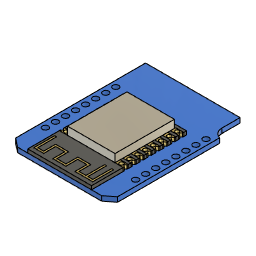
Wemos D1 Mini (Autodesk Fusion 360 design; units mm, degrees)
Autodesk Fusion 360 part; units mm, degrees
sketch "Sketch3" plane through (0, 0, 0) normal (0, 0, 1) x (1, 0, 0)
  line L0 (12.86, -17.28) -> (-12.86, -17.28)
  line L1 (-12.86, -17.28) -> (-12.86, 17.28)
  line L2 (-12.86, 17.28) -> (12.86, 17.28)
  line L3 (12.86, 17.28) -> (12.86, -17.28)
  line L4 (12.86, -17.28) -> (-12.86, 17.28) construction
  line L5 (-12.86, -17.28) -> (12.86, 17.28) construction
  line L6 (0, 55) -> (0, -53) construction
  line L7 (8.05, -17.28) -> (-8.05, -17.28)
  line L8 (-8.05, -17.28) -> (-8.05, 6.72)
  line L9 (-8.05, 6.72) -> (8.05, 6.72)
  line L10 (8.05, 6.72) -> (8.05, -17.28)
  line L11 (8.05, -17.28) -> (-8.05, 6.72) construction
  line L12 (-8.05, -17.28) -> (8.05, 6.72) construction
  line L13 (6, -9.28) -> (-6, -9.28)
  line L14 (-6, -9.28) -> (-6, 5.72)
  line L15 (6, 5.72) -> (6, -9.28)
  line L16 (6, -9.28) -> (-6, 5.72) construction
  line L17 (-6, -9.28) -> (6, 5.72) construction
  line L18 (-6, 5.72) -> (6, 5.72)
  line L19 (-9.2176, -9.28) -> (-6, -9.28) construction
  line L20 (-6, -7.98) -> (-8.05, -7.98)
  line L21 (-6, -9.28) -> (-8.05, -9.28)
  circle A0 centre (-6.9909, -8.6304) radius 0.5
  circle A1 centre (6.9909, -8.6304) radius 0.5
  line L22 (6, -9.28) -> (8.05, -9.28)
  line L23 (6, -7.98) -> (8.05, -7.98)
  arc A2 (8.05, -8.2791) -> (8.05, -8.9818) centre (8.05, -8.6304) ccw
  arc A3 (-8.05, -8.9818) -> (-8.05, -8.2791) centre (-8.05, -8.6304) ccw
  line L24 (-6, -5.98) -> (-8.05, -5.98)
  circle A4 centre (-6.9909, -6.6304) radius 0.5
  line L25 (-6, -7.28) -> (-8.05, -7.28)
  arc A5 (-8.05, -6.9818) -> (-8.05, -6.2791) centre (-8.05, -6.6304) ccw
  line L26 (6, -5.98) -> (8.05, -5.98)
  circle A6 centre (6.9909, -6.6304) radius 0.5
  arc A7 (8.05, -6.2791) -> (8.05, -6.9818) centre (8.05, -6.6304) ccw
  line L27 (6, -7.28) -> (8.05, -7.28)
  line L28 (-6, -3.98) -> (-8.05, -3.98)
  circle A8 centre (-6.9909, -4.6304) radius 0.5
  line L29 (-6, -5.28) -> (-8.05, -5.28)
  arc A9 (-8.05, -4.9818) -> (-8.05, -4.2791) centre (-8.05, -4.6304) ccw
  line L30 (6, -3.98) -> (8.05, -3.98)
  circle A10 centre (6.9909, -4.6304) radius 0.5
  arc A11 (8.05, -4.2791) -> (8.05, -4.9818) centre (8.05, -4.6304) ccw
  line L31 (6, -5.28) -> (8.05, -5.28)
  line L32 (-6, -1.98) -> (-8.05, -1.98)
  circle A12 centre (-6.9909, -2.6304) radius 0.5
  line L33 (-6, -3.28) -> (-8.05, -3.28)
  arc A13 (-8.05, -2.9818) -> (-8.05, -2.2791) centre (-8.05, -2.6304) ccw
  line L34 (6, -1.98) -> (8.05, -1.98)
  circle A14 centre (6.9909, -2.6304) radius 0.5
  arc A15 (8.05, -2.2791) -> (8.05, -2.9818) centre (8.05, -2.6304) ccw
  line L35 (6, -3.28) -> (8.05, -3.28)
  line L36 (-6, 0.02) -> (-8.05, 0.02)
  circle A16 centre (-6.9909, -0.6304) radius 0.5
  line L37 (-6, -1.28) -> (-8.05, -1.28)
  arc A17 (-8.05, -0.9818) -> (-8.05, -0.2791) centre (-8.05, -0.6304) ccw
  line L38 (6, 0.02) -> (8.05, 0.02)
  circle A18 centre (6.9909, -0.6304) radius 0.5
  arc A19 (8.05, -0.2791) -> (8.05, -0.9818) centre (8.05, -0.6304) ccw
  line L39 (6, -1.28) -> (8.05, -1.28)
  line L40 (-6, 2.02) -> (-8.05, 2.02)
  circle A20 centre (-6.9909, 1.3696) radius 0.5
  line L41 (-6, 0.72) -> (-8.05, 0.72)
  arc A21 (-8.05, 1.0182) -> (-8.05, 1.7209) centre (-8.05, 1.3696) ccw
  line L42 (6, 2.02) -> (8.05, 2.02)
  circle A22 centre (6.9909, 1.3696) radius 0.5
  arc A23 (8.05, 1.7209) -> (8.05, 1.0182) centre (8.05, 1.3696) ccw
  line L43 (6, 0.72) -> (8.05, 0.72)
  line L44 (-6, 4.02) -> (-8.05, 4.02)
  circle A24 centre (-6.9909, 3.3696) radius 0.5
  line L45 (-6, 2.72) -> (-8.05, 2.72)
  arc A25 (-8.05, 3.0182) -> (-8.05, 3.7209) centre (-8.05, 3.3696) ccw
  line L46 (6, 4.02) -> (8.05, 4.02)
  circle A26 centre (6.9909, 3.3696) radius 0.5
  arc A27 (8.05, 3.7209) -> (8.05, 3.0182) centre (8.05, 3.3696) ccw
  line L47 (6, 2.72) -> (8.05, 2.72)
  line L48 (-6, 6.02) -> (-8.05, 6.02)
  circle A28 centre (-6.9909, 5.3696) radius 0.5
  line L49 (-6, 4.72) -> (-8.05, 4.72)
  arc A29 (-8.05, 5.0182) -> (-8.05, 5.7209) centre (-8.05, 5.3696) ccw
  line L50 (6, 6.02) -> (8.05, 6.02)
  circle A30 centre (6.9909, 5.3696) radius 0.5
  arc A31 (8.05, 5.7209) -> (8.05, 5.0182) centre (8.05, 5.3696) ccw
  line L51 (6, 4.72) -> (8.05, 4.72)
  line L52 (-6, 5.72) -> (-6, 6.02)
  line L53 (6, 5.72) -> (6, 6.02)
  line L54 (5.1, -15.75) -> (5.1, -11)
  line L55 (-7.55, -11) -> (-7.55, -16.25)
  line L56 (-7.55, -16.25) -> (-5.05, -16.25)
  line L57 (-5.05, -16.25) -> (-5.05, -13.25)
  line L58 (-5.05, -13.25) -> (-2.75, -13.25)
  line L59 (-2.75, -13.25) -> (-2.75, -16.25)
  line L60 (-2.75, -16.25) -> (0.55, -16.25)
  line L61 (0.55, -16.25) -> (0.55, -13.25)
  line L62 (0.55, -13.25) -> (2.85, -13.25)
  line L63 (2.85, -13.25) -> (2.85, -16.25)
  line L64 (2.85, -16.25) -> (7.35, -16.25)
  line L65 (-7.05, -11) -> (-7.05, -15.75)
  line L66 (-7.05, -15.75) -> (-5.55, -15.75)
  line L67 (-5.55, -15.75) -> (-5.55, -12.75)
  line L68 (-5.55, -12.75) -> (-2.25, -12.75)
  line L69 (-2.25, -12.75) -> (-2.25, -15.75)
  line L70 (-2.25, -15.75) -> (0.05, -15.75)
  line L71 (0.05, -15.75) -> (0.05, -12.75)
  line L72 (0.05, -12.75) -> (3.35, -12.75)
  line L73 (3.35, -12.75) -> (3.35, -15.75)
  line L74 (3.35, -15.75) -> (5.1, -15.75)
  line L75 (-7.55, -11) -> (-7.05, -11)
  line L76 (7.35, -16.25) -> (7.35, -11)
  line L77 (5.6, -15.75) -> (6.85, -15.75)
  line L78 (6.85, -15.75) -> (6.85, -11)
  line L79 (5.6, -15.75) -> (5.6, -11)
  line L80 (5.1, -11) -> (5.6, -11)
  line L81 (6.85, -11) -> (7.35, -11)
  circle A32 centre (-11.36, 8.28) radius 0.75
  circle A33 centre (11.42, 8.28) radius 0.75
  circle A34 centre (-11.36, 5.74) radius 0.75
  circle A35 centre (11.42, 5.74) radius 0.75
  circle A36 centre (-11.36, 3.2) radius 0.75
  circle A37 centre (11.42, 3.2) radius 0.75
  circle A38 centre (-11.36, 0.66) radius 0.75
  circle A39 centre (11.42, 0.66) radius 0.75
  circle A40 centre (-11.36, -1.88) radius 0.75
  circle A41 centre (11.42, -1.88) radius 0.75
  circle A42 centre (-11.36, -4.42) radius 0.75
  circle A43 centre (11.42, -4.42) radius 0.75
  circle A44 centre (-11.36, -6.96) radius 0.75
  circle A45 centre (11.42, -6.96) radius 0.75
  circle A46 centre (-11.36, -9.5) radius 0.75
  circle A47 centre (11.42, -9.5) radius 0.75
  line L82 (11.01, 17.28) -> (11.01, 10.28)
  line L83 (11.01, 10.28) -> (12.86, 10.28)
  line L84 (10.61, -17.28) -> (12.86, -15.53)
  line L85 (-10.61, -17.28) -> (-12.86, -15.53)
  point P0 (0, -5.28)
  point P1 (0, -1.78)
  dimension "d14" = 25.72
  dimension "d15" = 34.56
  dimension "d16" = 24
  dimension "d17" = 16.1
  dimension "d18" = 15
  dimension "d19" = 12
  dimension "d21" = 1.3
  dimension "d22" = 1
  dimension "d23" = 1
  dimension "d26" = 0
  dimension "d27" = 14
  dimension "d42" = 0.5
  dimension "d43" = 1.5
  dimension "d44" = 9
  dimension "d45" = 1.5
  dimension "d48" = 22.78
  dimension "d49" = -2.54
  dimension "d50" = 7
  dimension "d51" = 1.85
  dimension "d52" = 2.25
  dimension "d53" = 1.75
  constraint perpendicular L0 L1
  constraint parallel L0 L2
  constraint parallel L1 L3
  constraint horizontal L0
  constraint coincident L4 origin
  constraint coincident L5 origin
  constraint perpendicular L2 L6
  constraint coincident origin L6
  constraint perpendicular L7 L8
  constraint parallel L7 L9
  constraint parallel L8 L10
  constraint horizontal L7
  constraint coincident L11 P0
  constraint coincident L12 P0
  constraint coincident L6 P0
  constraint collinear L0 L7
  constraint perpendicular L13 L14
  constraint parallel L14 L15
  constraint horizontal L13
  constraint coincident L16 P1
  constraint coincident L17 P1
  constraint coincident L6 P1
  constraint perpendicular L14 L19
  constraint coincident L14 L20.start
  constraint coincident L8 L20.end
  constraint perpendicular L8 L20
  constraint coincident L19 L21.end
  constraint coincident L8 L21.end
  constraint coincident L8 A3.centre
  constraint symmetric L6 L13.end L13.start
  constraint symmetric L6 L20.start L23.start
  constraint symmetric L6 L20.end L23.end
  constraint symmetric L6 L21.end L22.end
  constraint symmetric L6 A2 A3
  constraint symmetric L6 A0 A1
  constraint coincident L10 A2.end
  constraint coincident L10 A2.start
  constraint coincident L8 A3.end
  constraint coincident L8 A3.start
  constraint perpendicular L65 L75
  constraint perpendicular L79 L80
  constraint perpendicular L76 L81
  constraint coincident L2 L82.start
  constraint perpendicular L2 L82
  constraint coincident L3 L83.end
  constraint perpendicular L3 L83
  constraint coincident L0 L84.start
  constraint coincident L3 L84.end
  constraint symmetric L6 L84.start L85.start
  constraint symmetric L6 L84.end L85.end
  measures "d14" distance of L1.end L2.end
  measures "d15" distance of L0.end L1.end
  measures "d16" distance of L7.end L8.end
  measures "d17" distance of L8.end L9.end
  measures "d18" distance of L13.end L14.end
  measures "d19" distance of L14.end L15.start
  measures "d21" distance of L20 L21
  measures "d22" distance of L9 L18
  measures "d23" diameter of A0
  measures "d42" distance of L8 L55
  measures "d43" diameter of A32
  measures "d44" distance of L2 A32.centre
  measures "d45" distance of L1 A32.centre
  measures "d50" distance of L82.start L82.end
  measures "d51" distance of L82.end L83.end
  measures "d52" distance of L0.start L84.start
  measures "d53" distance of L0.start L84.end
extrude "Extrude6" add sketch "Sketch3" along normal blind 1.2 contours L0 L1 L2 L3 L8 L9 L10 L82 L83 L84 L85 | L0 L7 L8 L10 L13 L21 L22 | L10 L15 L22 L23 A2 | L8 L14 L20 L21 A3 | L10 A2 | L13 L14 L15 L18 | L8 A3 | L10 L15 L23 L27 | L8 L14 L20 L25 | L10 L15 L26 A7 L27 | L8 L14 L24 L25 A5 | L10 L15 L26 L31 | L8 L14 L24 L29 | L10 A7 | L10 L15 L30 A11 L31 | L8 A5 | L8 L14 L28 L29 A9 | L10 L15 L30 L35 | L8 L14 L28 L33 | L10 L15 L34 A15 L35 | L10 A11 | L8 L14 L32 L33 A13 | L8 A9 | L10 L15 L34 L39 | L8 L14 L32 L37 | L10 L15 L38 A19 L39 | L10 A15 | L8 L14 L36 L37 A17 | L8 A13 | L10 L15 L38 L43 | L8 L14 L36 L41 | L10 L15 L42 A23 L43 | L10 A19 | L8 L14 L40 L41 A21 | L8 A17 | L10 L15 L42 L47 | L8 L14 L40 L45 | L10 L15 L46 A27 L47 | L10 A23 | L8 L14 L44 L45 A25 | L8 A21 | L10 L15 L46 L51 | L8 L14 L44 L49 | L10 L15 L50 A31 L51 L53 | L10 A27 | L8 L14 L48 L49 A29 L52 | L8 A25 | L8 L9 L10 L18 L48 L50 L52 L53 | L10 A31 | L8 A29 | A0 | A1 | A4 | A6 | A8 | A10 | A12 | A14 | A16 | A18 | A20 | A22 | A24 | A26 | A28 | A30 | L54 L55 L56 L57 L58 L59 L60 L61 L62 L63 L64 L65 L66 L67 L68 L69 L70 L71 L72 L73 L74 L75 L76 L77 L78 L79 L80 L81 makes body 1
fillet "Fillet2" radius 2.5 1 edges at (11.01, 10.28, 0.6) on bodies 1
copy_body "Body->Comp1" bodies 1 removing the originals makes body 2 in component "PCB"
extrude "Extrude1" add sketch "Sketch3" along normal blind 0.9 from surface at 1.2 separate body contours L0 L7 L8 L10 L13 L21 L22 | L13 L14 L15 L18 | L10 L15 L23 L27 | L8 L14 L20 L25 | L10 L15 L26 L31 | L8 L14 L24 L29 | L10 L15 L30 L35 | L8 L14 L28 L33 | L10 L15 L34 L39 | L8 L14 L32 L37 | L10 L15 L38 L43 | L8 L14 L36 L41 | L10 L15 L42 L47 | L8 L14 L40 L45 | L10 L15 L46 L51 | L8 L14 L44 L49 | L8 L9 L10 L18 L48 L50 L52 L53 makes body 3 in component "8266"
extrude "Extrude2" add sketch "Sketch3" along normal up to surface (0.9 mm away) from surface at 1.2 separate body contours L10 L15 L22 L23 A2 | L8 L14 L20 L21 A3 | L10 L15 L26 A7 L27 | L8 L14 L24 L25 A5 | L10 L15 L30 A11 L31 | L8 L14 L28 L29 A9 | L10 L15 L34 A15 L35 | L8 L14 L32 L33 A13 | L10 L15 L38 A19 L39 | L8 L14 L36 L37 A17 | L10 L15 L42 A23 L43 | L8 L14 L40 L41 A21 | L10 L15 L46 A27 L47 | L8 L14 L44 L45 A25 | L10 L15 L50 A31 L51 L53 | L8 L14 L48 L49 A29 L52 | L54 L55 L56 L57 L58 L59 L60 L61 L62 L63 L64 L65 L66 L67 L68 L69 L70 L71 L72 L73 L74 L75 L76 L77 L78 L79 L80 L81 makes body 4 at (7.4885, 1.3198, 1.5) makes body 5 at (7.4885, -6.6802, 1.5) makes body 6 at (-6.4934, -4.6802, 1.5) makes body 7 at (-6.4934, 5.3198, 1.5) makes body 8 at (-6.4934, 1.3198, 1.5) makes body 9 at (-6.4934, -6.6802, 1.5) makes body 10 at (7.4885, -4.6802, 1.5) makes body 11 at (7.4885, 3.3198, 1.5) makes body 12 at (7.4885, -0.6802, 1.5) makes body 13 at (7.4885, -8.6802, 1.5) makes body 14 at (-6.4934, -2.6802, 1.5) makes body 15 at (-6.4934, 3.3198, 1.5) makes body 16 at (-6.4934, -0.6802, 1.5) makes body 17 at (-6.4934, -8.6802, 1.5) makes body 18 at (7.4885, -2.6802, 1.5) makes body 19 at (7.4885, 5.3198, 1.5) makes body 20 at (5.1, -16.0833, 1.2) in component "8266"
extrude "Extrude3" add sketch "Sketch3" along normal blind 2 from surface at 2.1 separate body contours L13 L14 L15 L18 makes body 21 in component "8266"
component "PCB" placed x (1, 0, 0) y (0, 1, 0) z (0, 0, 1) at (0, 0, 0)
component "8266" placed x (1, 0, 0) y (0, 1, 0) z (0, 0, 1) at (0, 0, 0)
equation "Width = 25.72 mm"
equation "Height = 34.56 mm"
equation "d14 = Width"
equation "d15 = Height"
